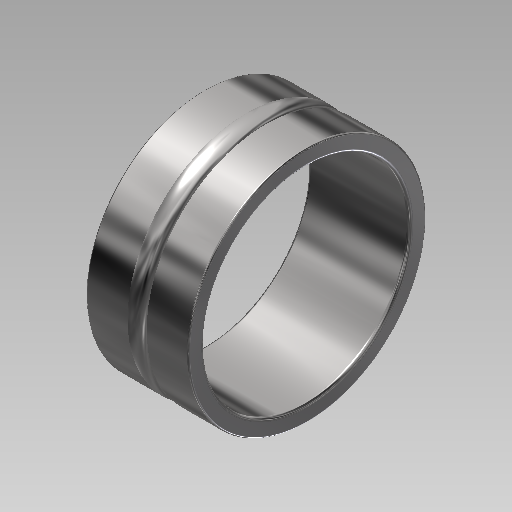
# Autodesk Inventor part: LF-1060ZZ_ir
Saved by Autodesk Inventor 2021 (Build 250183000, 183)
## iProperties
Created: 2019-09-04
Part Number: LF-1060ZZ_ir
Material: 鋼、炭素鋼
Catalog Web Link: www.cadenas.de
Description: Radial Flanged Ball Bearings (RF-Series/LF series) Metric ST ir-Radial Flanged Ball Bearings (RF-Series/LF series) Metric Shielded Type
Vendor: NMB
Document SubType Name: Modeling
Designer: psadmin
Manufacturer: NMB
Mass: 0.222198 g
Surface Area: 1.39162 cm^2
Volume: 0.0283055 cm^3
Density: 7.85 g/cm^3
Appearance: 半つや出し
Category: PARTsolutions
Company: NMB
PSOL_IDENT_0: {$CADENAS_DATA\23d-libs\nmb\pbbp\radial_flanged_ball_bearings\rfbb_rflfs_m\rflf_shielded_ir.prj},223
PSOL_IDENT_1: {VTYP=3D},{NB=LF-1060ZZ_ir},{LINA=LF-1060ZZ_ir},{NN=Radial Flanged Ball Bearings (RF-Series/LF seri
PSOL_IDENT_2: es) Metric ST ir},{DATE=11.11.2013 05:13:45},{GEOMDATE=24.10.2013 10:33:00},{VERSION=},{LINEID=1200}
PSOL_IDENT_3: ,{WBVAR=},{WBNUMERIC=}  {NB=LF-1060ZZ_ir},{LINA=LF-1060ZZ_ir},{KT=DUMMY},{IDNR=},{PN=LF-1060ZZ},{SHL
PSOL_IDENT_4: D=shielded},{FLANG=flanged},{SD=6.000},{D=10.000},{B=3.000},{SR=0.10},{BCZ=9},{DW=1.1906},{LI=6.95},
PSOL_IDENT_5: {LO=9.04},{D1=11.200},{C1=0.60},{D2=0.0},{C2=0.00},{COR=194},{CR=1029},{PCD=8.000},{U=9.191},{W=6.80
PSOL_IDENT_6: 9},{Y=0.595},{Z=0.595},{AA=9.072},{AC=0.60},{AD=0.000},{AF=0.00},{AQ=0.20},{AH=9.24},{AI=7.15},{AJ=0
PSOL_IDENT_7: .40}
NN: Radial Flanged Ball Bearings (RF-Series/LF series) Metric ST ir
NT: Radial Flanged Ball Bearings (RF-Series/LF series) Metric Shielded Type
NB: LF-1060ZZ_ir
NBSYN: $PN._ir
LINA: LF-1060ZZ_ir
PN: LF-1060ZZ
SHLD: shielded
FLANG: flanged
SD: 6
D: 10
B: 3
SR: 0.1
BCZ: 9
DW: 1.1906
LI: 6.95
LO: 9.04
D1: 0
C1: 0.6
D2: 0
C2: 0
COR: 194
CR: 1029
PCD: 8
U: 9.191
W: 6.809
Y: 0.595
Z: 0.595
AA: 9.072
AC: 0.6
AD: 0
AF: 0
AQ: 0.2
AH: 9.24
AI: 7.15
AJ: 0.4
SUPPLIER: NMB
ARTICLENO: LF-1060ZZ_ir
BOMINFO: LF-1060ZZ_ir
CREATOR: CADENAS GmbH
Title: LF-1060ZZ_ir
Author: Cadenas PARTsolutions
Comments: Radial Flanged Ball Bearings (RF-Series/LF series) Metric Shielded Type
Autodesk Inventor part; units mm, degrees
sketch "Sketch_5" plane through (0, 0, 0) normal (0, 0, 1) x (1, 0, 0)
  line L0 (3, 0) -> (0, 0)
  line L1 (0, 3.425) -> (0, 3.1)
  arc A0 (0, 3.1) -> (0.1, 3) centre (0.1, 3.1) ccw
  line L2 (0.1, 3) -> (2.9, 3)
  arc A1 (2.9, 3) -> (3, 3.1) centre (2.9, 3.1) ccw
  line L3 (3, 3.1) -> (3, 3.425)
  arc A2 (3, 3.425) -> (2.95, 3.475) centre (2.95, 3.425) ccw
  line L4 (2.95, 3.475) -> (1.7806, 3.475)
  arc A3 (1.2194, 3.475) -> (1.7806, 3.475) centre (1.5, 4) ccw
  line L5 (1.2194, 3.475) -> (0.05, 3.475)
  arc A4 (0.05, 3.475) -> (0, 3.425) centre (0.05, 3.425) ccw
  constraints: 12 end point, 10 point on circle, 5 centre point
revolve "Revolution1" add sketch "Sketch_5" angle 360 about axis through (3, 0, 0) along (1, 0, 0)
ref_plane "1_XY" through (1.5, 0, 0) normal (1, 0, 0) x (0, 0, -1)
ref_plane "1_YZ" through (1.5, 0, 0) normal (0, 0, -1) x (0, 1, 0)
ref_plane "1_ZX" through (1.5, 0, 0) normal (0, 1, 0) x (1, 0, 0)
ref_plane "Dummy_XY" through (0, 0, 0) normal (1, 0, 0) x (0, 0, -1)
ref_plane "Dummy_YZ" through (0, 0, 0) normal (0, 0, -1) x (0, 1, 0)
ref_plane "Dummy_ZX" through (0, 0, 0) normal (0, 1, 0) x (1, 0, 0)
ref_plane "shield1_XY" through (0.4, 0, 0) normal (1, 0, 0) x (0, 0, -1)
ref_plane "shield1_YZ" through (0.4, 0, 0) normal (0, 0, -1) x (0, 1, 0)
ref_plane "shield1_ZX" through (0.4, 0, 0) normal (0, 1, 0) x (1, 0, 0)
ref_plane "shield2_XY" through (2.6, 0, 0) normal (-1, 0, 0) x (0, 0, -1)
ref_plane "shield2_YZ" through (2.6, 0, 0) normal (0, 0, -1) x (0, -1, 0)
ref_plane "shield2_ZX" through (2.6, 0, 0) normal (0, -1, 0) x (-1, 0, 0)
body "Solid1"
